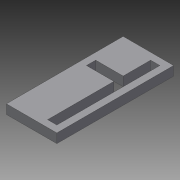
# Autodesk Inventor part: Carriage_Jig_Glue
Saved by Autodesk Inventor 2014 (Build 180170000, 170)
## iProperties
Created: 2014-10-17
Part Number: Carriage_Jig_Glue
Material: Generic
Document SubType Name: Modeling
Designer: ThatOtherGuy
Density: 1 g/cm^3
Appearance: Default
Author: ThatOtherGuy
Autodesk Inventor part; units mm, degrees
ref_plane "YZ Plane" through (0, 0, 0) normal (1, 0, 0) x (0, 1, 0)
ref_plane "XZ Plane" through (0, 0, 0) normal (0, 1, 0) x (-1, 0, 0)
ref_plane "XY Plane" through (0, 0, 0) normal (0, 0, 1) x (1, 0, 0)
sketch "Sketch1" plane through (0, 0, 0) normal (0, 0, 1) x (1, 0, 0)
  line L0 (0, 0) -> (36.731, 0)
  line L1 (36.731, 0) -> (36.731, 85)
  line L2 (36.731, 85) -> (0, 85)
  line L3 (0, 85) -> (0, 0)
  line L4 (25, 5) -> (25, 53.269)
  line L5 (25, 53.269) -> (5, 53.269)
  line L6 (5, 53.269) -> (5, 60)
  line L7 (5, 60) -> (25, 60)
  line L8 (25, 60) -> (25, 80)
  line L9 (25, 80) -> (31.731, 80)
  line L10 (31.731, 80) -> (31.731, 5)
  line L11 (31.731, 5) -> (25, 5)
  dimension "d1" = 75
  dimension "d2" = 20
  dimension "d3" = 6.731
  dimension "d4" = 20
  dimension "d7" = 5
  dimension "d8" = 5
  dimension "d9" = 5
  dimension "d10" = 5
  constraints: 24 end point, 7 parallel, 4 perpendicular, 2 collinear, 1 horizontal
  measures "d1" distance of L9.end L10.end
  measures "d2" distance between parallel lines of L9 L7
  measures "d3" distance of L8.end L9.end
  measures "d4" distance of L6.end L7.end
  measures "d7" distance between parallel lines of L6 L3
  measures "d8" distance between parallel lines of L0 L11
  measures "d9" distance between parallel lines of L2 L9
  measures "d10" distance between parallel lines of L1 L10
extrude "Extrusion1" add sketch "Sketch1" along normal blind 6.731
equation "\"d3\" = THICKB"
equation "\"d8\" = d7"
equation "\"d9\" = d7"
equation "\"d10\" = d7"
equation "\"d11\" = THICKB"
equation "\"THICKA\" = 3.175"
equation "\"THICKB\" = 6.731"
equation "\"THICKC\" = 12.7"
equation "\"MAGDIA\" = 9.5"
equation "\"BALLDIA\" = 12"
body "Solid1"
